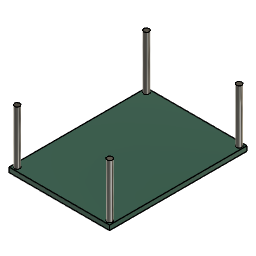
Final Prototype Model (Autodesk Fusion 360 archive; units mm, degrees)
design "pcb_sample_dim"
Autodesk Fusion 360 part; units mm, degrees
sketch "Sketch1" plane through (0, 0, 0) normal (0, 0, 1) x (1, 0, 0)
  line L0 (-17.5, 21.5) -> (19.8, 21.5)
  line L1 (19.8, 21.5) -> (19.8, -29.5)
  line L2 (19.8, -29.5) -> (-17.5, -29.5)
  line L3 (-17.5, -29.5) -> (-17.5, 21.5)
  dimension "d1" = 37.3
  dimension "d2" = 51
  dimension "d3" = 17.5
  dimension "d4" = 21.5
  constraint horizontal L0
  constraint vertical L1
  constraint horizontal L2
  constraint vertical L3
  measures "d1" distance of L0.start L0.end
  measures "d2" distance of L0.start L2.end
  measures "d3" horizontal distance of origin L2.end
  measures "d4" vertical distance of origin L0.start
extrude "Extrude1" add sketch "Sketch1" along normal blind 1.75 makes body 1
sketch "Sketch2" plane through (0, 0, 1.75) normal (0, 0, 1) x (-1, 0, 0)
  line L0 (17.5, 29.5) -> (-19.8, 29.5)
  line L1 (-19.8, 29.5) -> (-19.8, -21.5)
  line L2 (-19.8, -21.5) -> (17.5, -21.5)
  line L3 (17.5, -21.5) -> (17.5, 29.5)
  circle A0 centre (16, -20) radius 1
  circle A1 centre (-18.3948, -20) radius 1
  circle A2 centre (-18.3948, 28.0103) radius 1
  circle A3 centre (16, 28.0103) radius 1
  dimension "d7" = 2
  dimension "d8" = 2
  dimension "d9" = 2
  dimension "d10" = 2
  measures "d7" diameter of A1
  measures "d8" diameter of A2
  measures "d9" diameter of A3
  measures "d10" diameter of A0
extrude "Extrude2" add sketch "Sketch2" along normal blind 20 separate body contours A0 | A1 | A2 | A3 makes body 2 at (-16.7971, 19.3962, 15.0833) makes body 3 at (-16.9988, -27.9605, 15.0833) makes body 4 at (17.5977, 19.3962, 15.0833) makes body 5 at (17.8523, -28.8504, 15.0833)
